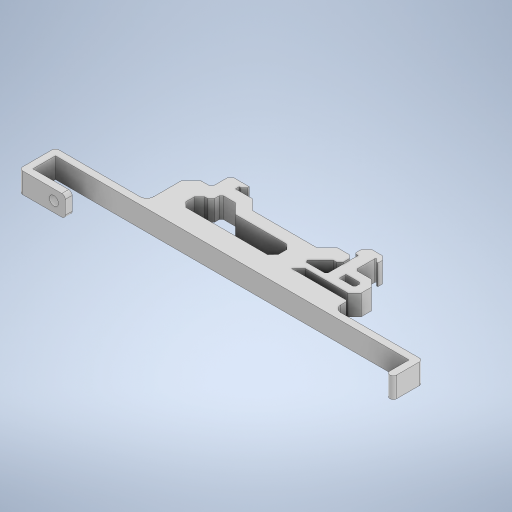
# Autodesk Inventor part: CO-1-01-jetsonMountSide2
Saved by Autodesk Inventor 2024 (Build 280153000, 153)
## iProperties
Created: 2023-11-22
Part Number: CO-1-01-jetsonMountSide2
Material: Generic
Document SubType Name: Modeling
Designer: t205b
Density: 1 g/cm^3
Appearance: Default
Author: t205b
Autodesk Inventor part; units mm, degrees
ref_plane "YZ Plane" through (0, 0, 0) normal (1, 0, 0) x (0, 1, 0)
ref_plane "XZ Plane" through (0, 0, 0) normal (0, 1, 0) x (-1, 0, 0)
ref_plane "XY Plane" through (0, 0, 0) normal (0, 0, 1) x (1, 0, 0)
sketch "Sketch1" plane through (0, 0, 0) normal (0, 1, 0) x (-1, 0, 0)
  line L0 (2, 8.6) -> (2, 2)
  line L1 (2, 2) -> (105.3, 2)
  line L2 (105.3, 2) -> (105.3, 8.6)
  line L3 (105.3, 8.6) -> (93.825, 8.6)
  line L4 (93.825, 8.6) -> (93.825, 10.6)
  line L5 (93.825, 10.6) -> (107.3, 10.6)
  line L6 (107.3, 10.6) -> (107.3, 0)
  line L7 (107.3, 0) -> (0, 0)
  line L8 (0, 0) -> (0, 8.6)
  line L9 (0, 8.6) -> (2, 8.6)
  dimension "d110" = 103.3
  dimension "d111" = 6.6
  dimension "d112" = 2
  dimension "d113" = 2
  dimension "d114" = 2
  dimension "d115" = 2
  dimension "d116" = 13.475
  dimension "d117" = 6.6
  constraints: 20 end point, 8 perpendicular, 1 coincident, 1 horizontal
  measures "d110" distance between parallel lines of L0 L2
  measures "d111" distance between parallel lines of L3 L1
  measures "d112" distance between parallel lines of L7 L1
  measures "d113" distance between parallel lines of L5 L3
  measures "d114" distance between parallel lines of L6 L2
  measures "d115" distance between parallel lines of L0 L8
  measures "d116" distance between parallel lines of L4 L6
  measures "d117" distance between parallel lines of L9 L1
extrude "Extrusion1" add sketch "Sketch1" along normal blind 6
sketch "Sketch2" plane through (107.3, 0, 10.6) normal (0, 0, -1) x (-1, 0, 0)
  line L0 (214.6, 0) -> (201.125, 0) projected
  line L1 (201.125, 0) -> (201.125, 6) projected
  line L2 (214.6, 6) -> (201.125, 6) projected
  line L3 (214.6, 0) -> (214.6, 6) projected
  circle A0 centre (204.45, 3) radius 1.325
  point P0 (107.3, 0)
  dimension "d118" = 2.65
  dimension "d119" = 10.15
  dimension "d120" = 6
  dimension "d121" = 3
  constraints: 1 centre point
  measures "d118" diameter of A0
  measures "d119" distance from line of A0.centre L3
  measures "d120" distance between parallel lines of L2 L0
  measures "d121" distance from line of A0.centre L2
extrude "Extrusion2" cut sketch "Sketch2" along normal blind 6 contours A0
fillet "Fillet3" radius 1 7 edges at (-93.825, 0, 9.6) (-93.825, 6, 9.6) (-107.3, 3, 10.6) (-107.3, 3, 0) (0, 3, 0) (0, 3, 8.6) (-2, 3, 8.6)
sketch "Sketch3" plane through (0, 0, 0) normal (0, -1, 0) x (1, 0, 0)
  line L0 (-62.6981, -12.9257) -> (-43.8067, -12.9257)
  line L1 (-77.6125, -12.9258) -> (-75.2261, -12.9258)
  line L2 (-79.0045, -11.5338) -> (-77.6125, -12.9258)
  line L3 (-80.5953, -9.9429) -> (-79.0045, -11.5338)
  line L4 (-42.0845, -8.4088) -> (-41.7933, -7.706)
  line L5 (-47.7839, -8.1194) -> (-49.2753, -9.4318)
  line L6 (-47.7839, -5.6476) -> (-49.2753, -3.9772)
  line L7 (-26.3093, 0) -> (-80.2, 0)
  line L8 (-26.3073, -3.9756) -> (-42.3153, -3.9756)
  line L9 (-74.6296, -7.9404) -> (-73.1382, -9.4319)
  line L10 (-26.3093, 0) -> (-25.91, -0.3973)
  line L11 (-25.91, -0.3973) -> (-25.91, -3.579)
  line L12 (-25.91, -3.579) -> (-26.3073, -3.9756)
  line L13 (-42.3153, -3.9756) -> (-40.3267, -5.9642)
  line L14 (-40.3267, -5.9642) -> (-27.8981, -5.9642)
  line L15 (-27.8981, -5.9642) -> (-25.9096, -7.9528)
  line L16 (-25.9096, -7.9528) -> (-25.9096, -10.9356)
  line L17 (-25.9096, -10.9356) -> (-27.8981, -12.9242)
  line L18 (-27.8981, -12.9242) -> (-32.1239, -12.9242)
  line L19 (-32.1239, -12.9242) -> (-32.621, -13.4213)
  line L20 (-32.621, -13.4213) -> (-32.621, -18.6613)
  line L21 (-32.621, -18.6613) -> (-32.3824, -18.8994)
  line L22 (-32.3824, -18.8994) -> (-31.4776, -17.9931)
  line L23 (-31.4776, -17.9931) -> (-31.0799, -17.9931)
  line L24 (-31.0799, -17.9931) -> (-31.0799, -19.2857)
  line L25 (-31.0799, -19.2857) -> (-32.273, -20.4809)
  line L26 (-32.273, -20.4809) -> (-35.3553, -20.4809)
  line L27 (-35.3553, -20.4809) -> (-36.8964, -18.9397)
  line L28 (-36.8964, -17.3489) -> (-36.8964, -18.9397)
  line L29 (-36.5484, -17.0009) -> (-35.8524, -17.0009)
  line L30 (-42.0845, -8.4088) -> (-38.3381, -12.1551)
  line L31 (-38.3381, -12.1551) -> (-37.3439, -12.1551)
  line L32 (-37.3439, -12.1551) -> (-36.3496, -13.1494)
  line L33 (-36.3496, -13.1494) -> (-36.3496, -14.9143)
  line L34 (-36.3496, -14.9143) -> (-37.3439, -15.9086)
  line L35 (-37.3439, -15.9086) -> (-40.8239, -15.9086)
  line L36 (-40.8239, -15.9086) -> (-43.8067, -12.9257)
  line L37 (-62.6981, -12.9257) -> (-65.681, -15.9086)
  line L38 (-65.681, -15.9086) -> (-70.6524, -15.9086)
  line L39 (-70.6524, -15.9086) -> (-70.6524, -17.0024)
  line L40 (-70.6524, -17.0024) -> (-70.1554, -17.0024)
  line L41 (-70.1554, -17.0024) -> (-69.161, -17.9967)
  line L42 (-69.161, -17.9967) -> (-69.161, -18.4938)
  line L43 (-69.161, -18.4938) -> (-73.6353, -18.4938)
  line L44 (-73.6353, -18.4938) -> (-74.6296, -17.4995)
  line L45 (-74.6296, -17.4995) -> (-74.6296, -13.5224)
  line L46 (-74.6296, -13.5224) -> (-75.2261, -12.9258)
  line L47 (-80.5953, -9.9429) -> (-80.5953, -0.3979)
  line L48 (-80.5953, -0.3979) -> (-80.2, 0)
  line L49 (-74.6296, -7.9404) -> (-74.6296, -5.4687)
  line L50 (-74.6296, -5.4687) -> (-73.1382, -3.9772)
  line L51 (-73.1382, -3.9772) -> (-49.2753, -3.9772)
  line L52 (-47.7839, -5.6476) -> (-47.7839, -8.1194)
  line L53 (-49.2753, -9.4318) -> (-64.1454, -9.4318)
  line L54 (-67.1282, -12.4147) -> (-70.6524, -12.4147)
  line L55 (-71.2491, -10.4261) -> (-72.2433, -9.4319)
  line L56 (-71.2491, -11.8181) -> (-71.2491, -10.4261)
  line L57 (-72.2433, -9.4319) -> (-73.1382, -9.4319)
  line L58 (-70.6524, -12.4147) -> (-71.2491, -11.8181)
  line L59 (-64.1454, -9.4318) -> (-67.1282, -12.4147)
  line L60 (-32.856, -10.425) -> (-32.856, -8.4638)
  line L61 (-32.856, -8.4638) -> (-28.9062, -8.4638)
  line L62 (-28.9062, -8.4638) -> (-28.4091, -8.9609)
  line L63 (-28.4091, -8.9609) -> (-28.4091, -9.9278)
  line L64 (-28.4091, -9.9278) -> (-28.9062, -10.425)
  line L65 (-28.9062, -10.425) -> (-32.856, -10.425)
  line L66 (-36.5484, -17.0009) -> (-36.8964, -17.3489)
  line L67 (-35.8524, -8.2031) -> (-35.8524, -17.0009)
  line L68 (-36.3496, -7.706) -> (-35.8524, -8.2031)
  line L69 (-36.3496, -7.706) -> (-41.7933, -7.706)
  line L70 (-1, 0) -> (-106.3, 0) projected
  line L71 (-107.3, 1) -> (-107.3, 9.6) projected
  line L72 (0, 7.6) -> (0, 1) projected
  point P0 (0, 0)
  point P1 (-74.6296, -6.7046)
  dimension "d18" = 9.545
  dimension "d19" = 3.9771
  dimension "d20" = 4.4743
  dimension "d21" = 4.9714
  dimension "d22" = 3.5242
  dimension "d23" = 2.9829
  dimension "d24" = 0.9943
  dimension "d25" = 0.398
  dimension "d26" = 53.8907
  dimension "d27" = 2.4718
  dimension "d28" = 1.4914
  dimension "d29" = 1.4914
  dimension "d30" = 1.392
  dimension "d31" = 0.5966
  dimension "d32" = 23.8629
  dimension "d33" = 1.4914
  dimension "d34" = 2.4718
  dimension "d35" = 14.8701
  dimension "d36" = 2.9829
  dimension "d37" = 18.8914
  dimension "d38" = 2.9829
  dimension "d39" = 2.9829
  dimension "d40" = 3.48
  dimension "d41" = 3.7464
  dimension "d42" = 0.7028
  dimension "d43" = 5.4437
  dimension "d44" = 8.7978
  dimension "d45" = 0.4971
  dimension "d46" = 1.5909
  dimension "d47" = 0.348
  dimension "d48" = 0.696
  dimension "d49" = 1.5411
  dimension "d50" = 3.0823
  dimension "d51" = 1.1931
  dimension "d52" = 1.2927
  dimension "d53" = 0.3977
  dimension "d54" = 0.9048
  dimension "d55" = 0.2386
  dimension "d56" = 5.24
  dimension "d57" = 0.4971
  dimension "d58" = 4.2257
  dimension "d59" = 1.9886
  dimension "d60" = 2.9829
  dimension "d61" = 1.9886
  dimension "d62" = 12.4286
  dimension "d63" = 1.9886
  dimension "d64" = 16.008
  dimension "d65" = 0.3973
  dimension "d66" = 3.1817
  dimension "d67" = 2.9829
  dimension "d68" = 2.9829
  dimension "d69" = 2.9829
  dimension "d70" = 0.9943
  dimension "d71" = 0.9943
  dimension "d72" = 0.9943
  dimension "d73" = 3.7463
  dimension "d74" = 1.7649
  dimension "d75" = 0.9943
  dimension "d76" = 0.9943
  dimension "d77" = 0.4971
  dimension "d78" = 0.4971
  dimension "d79" = 0.4971
  dimension "d80" = 0.4971
  dimension "d81" = 0.4971
  constraints: 140 end point, 26 parallel, 17 perpendicular, 2 vertical, 1 collinear, 1 midpoint
  measures "d18" distance of L47.end L3.start
  measures "d19" distance of L46.start L45.start
  measures "d20" distance of L43.end L42.end
  measures "d21" distance of L39.start L38.start
  measures "d22" distance of L54.start L58.start
  measures "d23" horizontal distance of L1.start L3.start
  measures "d24" horizontal distance of L45.start L43.end
  measures "d25" vertical distance of L7.end L47.end
  measures "d26" distance of L7.start L7.end
  measures "d27" distance of L9.start L49.end
  measures "d28" horizontal distance of L49.end L51.start
  measures "d29" horizontal distance of L9.start L9.end
  measures "d30" distance of L58.end L56.end
  measures "d31" vertical distance of L58.start L58.end
  measures "d32" distance of L51.start L51.end
  measures "d33" horizontal distance of L6.start L51.end
  measures "d34" distance of L6.start L5.start
  measures "d35" distance of L53.start L53.end
  measures "d36" horizontal distance of L53.end L54.start
  measures "d37" distance of L0.end L0.start
  measures "d38" horizontal distance of L38.start L0.start
  measures "d39" horizontal distance of L0.end L35.end
  measures "d40" distance of L35.end L34.end
  measures "d41" horizontal distance of L31.start L4.start
  measures "d42" vertical distance of L4.start L4.end
  measures "d43" distance of L4.end L68.start
  measures "d44" distance of L68.end L67.end
  measures "d45" horizontal distance of L68.start L68.end
  measures "d46" distance of L66.end L28.end
  measures "d47" horizontal distance of L66.end L29.start
  measures "d48" distance of L67.end L29.start
  measures "d49" horizontal distance of L28.end L27.start
  measures "d50" distance of L27.start L26.start
  measures "d51" horizontal distance of L26.start L24.end
  measures "d52" distance of L24.end L24.start
  measures "d53" distance of L24.start L22.end
  measures "d54" horizontal distance of L22.end L22.start
  measures "d55" horizontal distance of L22.start L20.end
  measures "d56" distance of L20.end L20.start
  measures "d57" horizontal distance of L20.start L19.start
  measures "d58" distance of L19.start L18.start
  measures "d59" horizontal distance of L16.end L18.start
  measures "d60" distance of L15.end L16.end
  measures "d61" horizontal distance of L14.end L15.end
  measures "d62" distance of L14.end L13.end
  measures "d63" horizontal distance of L13.start L13.end
  measures "d64" distance of L13.start L8.start
  measures "d65" horizontal distance of L8.start L11.end
  measures "d66" distance of L11.end L10.end
  measures "d67" horizontal distance of L38.start L0.start
  measures "d68" horizontal distance of L53.end L54.start
  measures "d69" horizontal distance of L0.end L35.end
  measures "d70" horizontal distance of L32.end L31.end
  measures "d71" horizontal distance of L32.end L31.end
  measures "d72" distance of L31.end L31.start
  measures "d73" vertical distance of L31.start L4.start
  measures "d74" distance of L34.start L32.end
  measures "d75" horizontal distance of L34.end L34.start
  measures "d76" horizontal distance of L34.end L34.start
  measures "d77" horizontal distance of L20.start L19.start
  measures "d78" horizontal distance of L63.end L65.start
  measures "d79" horizontal distance of L63.end L65.start
  measures "d80" horizontal distance of L61.end L62.end
  measures "d81" horizontal distance of L61.end L62.end
extrude "Extrusion3" add sketch "Sketch3" against normal blind 6
fillet "Fillet4" radius 2 4 edges at (-25.91, 3, -0.3973) (-26.3093, 3, 0) (-80.5953, 3, -0.3979) (-80.2, 3, 0)
body "Solid1"
